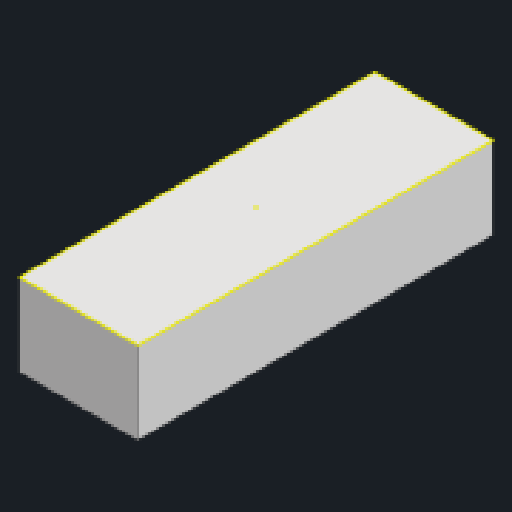
# Autodesk Inventor part: bigLipo
Saved by Autodesk Inventor 2023 (Build 270158000, 158)
## iProperties
Created: 2024-04-13
Part Number: bigLipo
Material: Generic
Document SubType Name: Modeling
Designer: szymo
Density: 1 g/cm^3
Appearance: Default
Author: szymo
Autodesk Inventor part; units mm, degrees
ref_plane "YZ Plane" through (0, 0, 0) normal (1, 0, 0) x (0, 1, 0)
ref_plane "XZ Plane" through (0, 0, 0) normal (0, 1, 0) x (-1, 0, 0)
ref_plane "XY Plane" through (0, 0, 0) normal (0, 0, 1) x (1, 0, 0)
sketch "Sketch1" plane through (0, 0, 0) normal (0, 1, 0) x (-1, 0, 0)
  line L0 (11.5, 34.5) -> (-11.5, 34.5)
  line L1 (-11.5, 34.5) -> (-11.5, -34.5)
  line L2 (-11.5, -34.5) -> (11.5, -34.5)
  line L3 (11.5, -34.5) -> (11.5, 34.5)
  line L4 (11.5, 34.5) -> (-11.5, -34.5) construction
  line L5 (-11.5, 34.5) -> (11.5, -34.5) construction
  point P0 (0, 0)
  dimension "d0" = 23
  dimension "d1" = 69
  constraints: 12 end point, 2 midpoint, 2 parallel, 1 horizontal, 1 perpendicular
  measures "d0" distance of L2.end L1.end
  measures "d1" distance of L1.end L0.end
extrude "Extrusion1" add sketch "Sketch1" along normal blind 16
sketch "Sketch3" plane through (11.5, 0, 34.5) normal (1, 0, 0) x (0, 0, -1)
  line L0 (0, 0) -> (69, 0) projected
  line L1 (69, 0) -> (69, 16) projected
  line L2 (0, 16) -> (69, 16) projected
  line L3 (0, 0) -> (0, 16) projected
  line L4 (41.4, 13.119) -> (36.4, 13.119) projected
  line L5 (36.4, 13.119) -> (36.4, 11.6808) projected
  line L6 (36.4, 11.6668) -> (36.4, 3.375) projected
  line L7 (41.4, 2.875) -> (36.4, 2.875) projected
  line L8 (36.4, 3.375) -> (36.4, 2.875) projected
  line L9 (0, 0) -> (0, 16) projected
  line L10 (36.4, 13.119) -> (0, 13.119)
  line L11 (0, 13.119) -> (0, 2.875)
  line L12 (0, 2.875) -> (36.4, 2.875)
  line L13 (36.4, 2.875) -> (36.4, 13.119)
  point P0 (34.5, 0)
  constraints: 8 end point, 2 parallel, 1 horizontal, 1 perpendicular, 1 point on line
ref_plane "Work Plane1" through (16.75, 3.375, -6.9) normal (1, 0, 0) x (0, 1, 0)
extrude "Extrusion2" add sketch "Sketch3" along normal up to surface (5.25 mm away) contours L3 L10 L5 L13 L6 L8 L12
body "Solid1"
